Fixation Nema14 (Autodesk Fusion 360 design; units mm, degrees)
Autodesk Fusion 360 part; units mm, degrees
note: some values were not read from the file. Chosen so that the rebuilt part matches the saved one: which face or edge a step refers to; which pieces of a blend or face edit are solid. Set by a fixed rule: which sketch regions a step uses.
sketch "Sketch1" plane through (0, 0, 0) normal (0, 0, 1) x (-1, 0, 0)
  circle A0 centre (13, -13) radius 2
  circle A1 centre (-13, -13) radius 2
  line L0 (17, 15.2929) -> (15.2929, 17)
  line L1 (15.2929, 17) -> (-15.2929, 17)
  line L2 (-15.2929, 17) -> (-17, 15.2929)
  line L3 (-17, 15.2929) -> (-17, -15.2929)
  line L4 (-17, -15.2929) -> (-15.2929, -17)
  line L5 (-15.2929, -17) -> (15.2929, -17)
  line L6 (15.2929, -17) -> (17, -15.2929)
  circle A2 centre (0, 0) radius 11.5
  circle A3 centre (-13, 13) radius 2
  circle A4 centre (13, 13) radius 2
  circle A5 centre (13, -13) radius 1.6
  circle A6 centre (13, 13) radius 1.6
  line L7 (0, 0) -> (17.5, 0) construction
  line L8 (13.0004, -11.4) -> (13, 13) construction
  line L9 (9, 17) -> (13.0002, 0.335) construction
  arc A7 (9, -8.6747) -> (9, 8.6747) centre (0, 0) ccw
  line L10 (9, 17) -> (9, 8.6747)
  line L11 (9, -8.6747) -> (9, -17)
  line L12 (13.0002, 0.335) -> (9, -17) construction
  line L13 (17.5, -17.5) -> (17.5, 17.5)
  line L14 (17.5, 0) -> (17.5, -14.8)
  line L15 (17.5, 0) -> (17.5, 14.8)
  line L16 (9, -17) -> (15.3, -17)
  line L17 (9, 17) -> (15.3, 17)
  line L18 (17.5, 14.8) -> (15.3, 17)
  line L19 (15.3, -17) -> (17.5, -14.8)
  line L20 (9, -17) -> (9, 17) construction
  point P0 (13, 13)
  dimension "d1" = 3.2
  dimension "d2" = 3.2
  dimension "d4" = 12.5
  dimension "d5" = 8.3253
  dimension "d6" = 8.3253
  dimension "d15" = 14.8
  dimension "d16" = 14.8
  dimension "d20" = 135
  dimension "d21" = 135
  dimension "d33" = 4.5
  constraint concentric A0 A5
  constraint concentric A4 A6
  constraint coincident A2.centre L7.start
  constraint coincident P0 A4.centre
  constraint coincident A5 L8.start
  constraint coincident L8 L9.end
  constraint coincident A7.start L10
  constraint collinear L10 L11
  constraint perpendicular L7 L14
  constraint perpendicular L7 L15
  constraint coincident L7.end L13
  constraint horizontal L7
  constraint perpendicular L13 L16
  constraint perpendicular L13 L17
  constraint coincident L1 L17.end
  constraint perpendicular L17 L20
  measures "d1" diameter of A5
  measures "d2" diameter of A6
  measures "d4" radius of A7
  measures "d5" distance of L11.end A7.start
  measures "d6" distance of L9.start A7.end
  measures "d15" distance of L7.end L14.end
  measures "d16" distance of L7.end L15.end
  measures "d20" angle of L15 L18
  measures "d21" angle of L14 L19
  measures "d33" distance of L15 P0
extrude "Extrude1" add sketch "Sketch1" along normal blind 3 contours L1 L5 A7 L10 L11 L13 L14 L15 L16 L17 L18 L19
sketch "Sketch3" plane through (-17.5, 0, 0) normal (-1, 0, 0) x (0, -1, 0)
  circle A0 centre (0, 1.5) radius 4.05
  circle A1 centre (0, 1.5) radius 5.05
  line L0 (-14.8, 0) -> (14.8, 0)
  line L1 (14.8, 0) -> (14.8, 3)
  line L2 (14.8, 3) -> (-14.8, 3)
  line L3 (-14.8, 3) -> (-14.8, 0)
  line L4 (0, 3) -> (0, 0) construction
  line L5 (-3.762, 0) -> (3.762, 0)
  dimension "d22" = 8.1
  dimension "d25" = 1
  constraint midpoint L2 L4.start
  constraint coincident L4.end origin
  constraint midpoint A0.centre L4
  constraint coincident A0 L5.start
  constraint coincident L0 L5.start
  constraint coincident A0 L5.end
  constraint coincident L0 L5.end
  measures "d22" diameter of A0
extrude "Extrude2" add sketch "Sketch3" along normal blind 8 contours A0 L0 L5 | A0 L0 L2 L5 | A0 L2
extrude "Extrude3" add sketch "Sketch3" along normal blind 0.5 contours A0 A1 L0 L2 | A0 A1 L0 L2
extrude "Extrude4" add sketch "Sketch3" against normal blind 5 contours A0 L0 L2 L5 | A0 L2
fillet "Fillet1" radius 12.5 2 edges at (-15.25, 3.762, 3) (-15.25, -3.762, 3)
named bodies: "Fixation Nema14"
